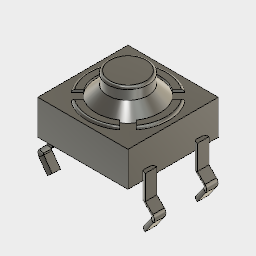
3101 8mm soft button (Autodesk Fusion 360 design; units mm, degrees)
Autodesk Fusion 360 part; units mm, degrees
sketch "Sketch1" plane through (0, 0, 0) normal (0, 0, 1) x (1, 0, 0)
  line L0 (3.9, -3.9) -> (-3.9, -3.9)
  line L1 (-3.9, -3.9) -> (-3.9, 3.9)
  line L2 (-3.9, 3.9) -> (3.9, 3.9)
  line L3 (3.9, 3.9) -> (3.9, -3.9)
  line L4 (3.9, -3.9) -> (-3.9, 3.9) construction
  line L5 (-3.9, -3.9) -> (3.9, 3.9) construction
  circle A0 centre (0, 0) radius 1.75
  line L6 (0, 0) -> (0, 5) construction
  line L7 (0, 0) -> (5, 0) construction
  line L8 (-4.25, 1.75) -> (-4.25, 2.75)
  arc A1 (-3.9, 2.6071) -> (-4.25, 2.75) centre (-4.25, 2.25) ccw
  arc A2 (-4.25, 1.75) -> (-3.9, 1.8929) centre (-4.25, 2.25) ccw
  arc A3 (4.25, 2.75) -> (3.9, 2.6071) centre (4.25, 2.25) ccw
  line L9 (4.25, 1.75) -> (4.25, 2.75)
  arc A4 (3.9, 1.8929) -> (4.25, 1.75) centre (4.25, 2.25) ccw
  arc A5 (4.25, -1.75) -> (3.9, -1.8929) centre (4.25, -2.25) ccw
  line L10 (4.25, -1.75) -> (4.25, -2.75)
  arc A6 (3.9, -2.6071) -> (4.25, -2.75) centre (4.25, -2.25) ccw
  line L11 (-4.25, -1.75) -> (-4.25, -2.75)
  arc A7 (-3.9, -1.8929) -> (-4.25, -1.75) centre (-4.25, -2.25) ccw
  arc A8 (-4.25, -2.75) -> (-3.9, -2.6071) centre (-4.25, -2.25) ccw
  dimension "d1" = 7.8
  dimension "d2" = 7.8
  dimension "d3" = 3.5
  dimension "d4" = 1
  dimension "d5" = 4.25
  dimension "d6" = 2.25
  measures "d1" distance of L0.end L1.end
  measures "d2" distance of L1.end L2.end
  measures "d3" diameter of A0
  measures "d4" diameter of A1
  measures "d5" distance of A1.centre L6
  measures "d6" distance of A1.centre L7
extrude "Extrude1" add sketch "Sketch1" along normal blind 3 contours L0 L1 L2 L3 | A0 makes body 1
sketch "Sketch2" plane through (0, 0, 0) normal (0, 1, 0) x (1, 0, 0)
  line L0 (3.9, 0) -> (4.25, 0)
  line L1 (4.075, 0) -> (4.075, -0.2) construction
  line L2 (4.075, 0) -> (4.075, 1.375)
  line L3 (0, 0) -> (4.95, 0)
  line L4 (4.7719, 2.0714) -> (4.075, 1.375)
  line L5 (4.8057, 2.4556) -> (4.075, 3.5)
  arc A0 (4.7719, 2.0714) -> (4.8057, 2.4556) centre (4.5599, 2.2836) ccw
  dimension "d11" = 3.5
  dimension "d12" = 4.95
  dimension "d13" = 100
  dimension "d14" = 0.3
  measures "d11" distance of L1.start L5.end
  measures "d12" distance of L3.start L3.end
  measures "d13" angle of L4 L5
  measures "d14" radius of A0
sweep "Sweep1" add profiles "Sketch1" path "Sketch2" along L2 L4 A0 L5 section 1 contours L3 A5 L10 A6 | L3 A3 L9 A4 separate body makes body 2 at (4.25, -2.4167, -0.8683) makes body 3 at (4.25, 2.0833, -0.8683)
extrude "Extrude3" add sketch "Sketch1" along normal blind 0.8 contours L3 A5 L10 A6 | L3 A3 L9 A4 bodies 2 3
mirror "Mirror1" about plane through (0, 0, 0) normal (1, 0, 0) of bodies 2 3 makes body 4 at (-4.25, 2.0833, -0.6017) makes body 5 at (-4.25, -2.0833, -0.6017)
sketch "Sketch3" plane through (0, 0, 3) normal (0, 0, 1) x (-1, 0, 0)
  line L0 (-3.9, -3.9) -> (3.9, -3.9)
  line L1 (3.9, -3.9) -> (3.9, 3.9)
  line L2 (3.9, 3.9) -> (-3.9, 3.9)
  line L3 (-3.9, 3.9) -> (-3.9, -3.9)
  circle A0 centre (0, 0) radius 1.75
  dimension "d24" = 3.5
  measures "d24" diameter of A0
extrude "Extrude4" add sketch "Sketch3" along normal blind 2 contours A0 bodies 1
chamfer "Chamfer1" distance 1 angle 45 1 edges at (1.6316, -0.6328, 3) on bodies 1
sketch "Sketch4" plane through (0, 0, 3) normal (0, 0, 1) x (-1, 0, 0)
  line L0 (-3.9, -3.9) -> (3.9, -3.9)
  line L1 (3.9, -3.9) -> (3.9, 3.9)
  line L2 (3.9, 3.9) -> (-3.9, 3.9)
  line L3 (-3.9, 3.9) -> (-3.9, -3.9)
  circle A0 centre (0, 0) radius 2.75
  circle A1 centre (0, 0) radius 3.5
  line L4 (3.5355, -2.8284) -> (2.8284, -3.5355)
  line L5 (2.8284, -3.5355) -> (-3.5355, 2.8284)
  line L6 (-3.5355, 2.8284) -> (-2.8284, 3.5355)
  line L7 (-2.8284, 3.5355) -> (3.5355, -2.8284)
  line L8 (0, 0) -> (0, -4.8) construction
  line L9 (2.8284, 3.5355) -> (-3.5355, -2.8284)
  line L10 (-3.5355, -2.8284) -> (-2.8284, -3.5355)
  line L11 (-2.8284, -3.5355) -> (3.5355, 2.8284)
  line L12 (3.5355, 2.8284) -> (2.8284, 3.5355)
  dimension "d28" = 0.75
  dimension "d32" = 1
  measures "d32" distance of L4.start L4.end
extrude "Extrude5" add sketch "Sketch4" along normal blind 0.2 contours A0 A1 L7 L11 | A0 A1 L7 L9 | A0 A1 L5 L11 | A0 A1 L5 L9 bodies 1
fillet "Fillet1" radius 0.2 1 edges at (1.6316, 0.6328, 5) on bodies 1
fillet "Fillet2" radius 0.2 4 edges at (0, 3.5, 3.2) (3.5, 0, 3.2) (0, -3.5, 3.2) (-3.5, 0, 3.2) on bodies 1
equation "d12 = ( 9.9 / 2 ) * 1 mm"
